Autodesk Inventor part; units mm, degrees
(part 2 of 2)
  arc A608 (10.5835, 25.1123) -> (10.4066, 24.8539) centre (14.8434, 22.0065) ccw
  arc A609 (10.8252, 25.4234) -> (10.5835, 25.1123) centre (15.7615, 21.3378) ccw
  arc A610 (11.147, 25.7878) -> (10.8252, 25.4234) centre (16.6706, 20.5861) ccw
  arc A611 (9.9958, 26.1618) -> (9.6113, 26.2702) centre (4.2393, 6.4866) ccw
  arc A612 (10.0419, 25.6779) -> (9.9958, 26.1618) centre (2.4697, 25.2002) ccw
  arc A613 (10.0547, 25.2841) -> (10.0419, 25.6779) centre (3.647, 25.2741) ccw
  arc A614 (10.4066, 24.8539) -> (10.0459, 24.9711) centre (4.2393, 6.4866) ccw
  arc A615 (10.0459, 24.9711) -> (10.0547, 25.2841) centre (4.7827, 25.2754) ccw
  arc A616 (9.1026, 25.5526) -> (8.9465, 25.2811) centre (13.5931, 22.7906) ccw
  arc A617 (9.3192, 25.8817) -> (9.1026, 25.5526) centre (14.5608, 22.1961) ccw
  arc A618 (9.6113, 26.2702) -> (9.3192, 25.8817) centre (15.526, 21.5179) ccw
  arc A619 (8.4344, 26.5528) -> (8.0426, 26.6307) centre (4.2393, 6.4866) ccw
  arc A620 (8.5183, 26.074) -> (8.4344, 26.5528) centre (1.0069, 25.0037) ccw
  arc A621 (8.5619, 25.6824) -> (8.5183, 26.074) centre (2.1747, 25.1697) ccw
  arc A622 (8.9465, 25.2811) -> (8.5777, 25.3697) centre (4.2393, 6.4866) ccw
  arc A623 (8.5777, 25.3697) -> (8.5619, 25.6824) centre (3.3069, 25.2601) ccw
  arc A624 (7.5917, 25.8754) -> (7.4574, 25.5925) centre (12.285, 23.4742) ccw
  arc A625 (7.7818, 26.2205) -> (7.5917, 25.8754) centre (13.2964, 22.9575) ccw
  arc A626 (8.0426, 26.6307) -> (7.7818, 26.2205) centre (14.3119, 22.3571) ccw
  arc A627 (6.8471, 26.8201) -> (6.4504, 26.867) centre (4.2393, 6.4866) ccw
  arc A628 (6.9683, 26.3493) -> (6.8471, 26.8201) centre (-0.436, 24.693) ccw
  arc A629 (7.0425, 25.9624) -> (6.9683, 26.3493) centre (0.7152, 24.9501) ccw
  arc A630 (7.4574, 25.5925) -> (7.0828, 25.6518) centre (4.2393, 6.4866) ccw
  arc A631 (7.0828, 25.6518) -> (7.0425, 25.9624) centre (1.8368, 25.1291) ccw
  arc A632 (6.0601, 26.0787) -> (5.9484, 25.7861) centre (10.9274, 24.0531) ccw
  arc A633 (6.2226, 26.4376) -> (6.0601, 26.0787) centre (11.9762, 23.6173) ccw
  arc A634 (6.4504, 26.867) -> (6.2226, 26.4376) centre (13.0356, 23.0985) ccw
  arc A635 (5.2437, 26.962) -> (4.8445, 26.9777) centre (4.2393, 6.4866) ccw
  arc A636 (5.4015, 26.5022) -> (5.2437, 26.962) centre (-1.85, 24.27) ccw
  arc A637 (5.5058, 26.1223) -> (5.4015, 26.5022) centre (-0.7225, 24.6167) ccw
  arc A638 (5.9484, 25.7861) -> (5.5703, 25.8158) centre (4.2393, 6.4866) ccw
  arc A639 (5.5703, 25.8158) -> (5.5058, 26.1223) centre (0.3816, 24.8831) ccw
  circle A640 centre (4.2393, 6.4866) radius 18.25
  circle A641 centre (4.2393, 6.4866) radius 6
  circle A642 centre (4.2393, 6.4866) radius 20.5 construction
  circle A643 centre (4.2393, 6.4866) radius 2
  line L0 (4.2393, 6.4866) -> (-6.2776, -1.9776)
  circle A644 centre (-6.2776, -1.9776) radius 1.5
  circle A645 centre (-6.2776, -1.9776) radius 3.5
  circle A646 centre (4.2393, 6.4866) radius 4
  circle A647 centre (12.7036, -4.0303) radius 1.5
  circle A648 centre (12.7036, -4.0303) radius 3.5
  circle A649 centre (14.7563, 14.9509) radius 1.5
  circle A650 centre (14.7563, 14.9509) radius 3.5
  circle A651 centre (-4.225, 17.0036) radius 1.5
  circle A652 centre (-4.225, 17.0036) radius 3.5
  point P0 (0, 0)
  point P1 (0, 0)
  point P2 (4.2393, 28.9866)
  point P3 (2.474, 28.9173)
  point P4 (0.7195, 28.7096)
  point P5 (-1.0132, 28.3649)
  point P6 (-2.7136, 27.8854)
  point P7 (-4.3711, 27.2739)
  point P8 (-5.9755, 26.5343)
  point P9 (-7.5169, 25.671)
  point P10 (-8.9859, 24.6895)
  point P11 (-10.3733, 23.5958)
  point P12 (-11.6706, 22.3965)
  point P13 (-12.8698, 21.0992)
  point P14 (-13.9636, 19.7118)
  point P15 (-14.9451, 18.2428)
  point P16 (-15.8083, 16.7014)
  point P17 (-16.548, 15.097)
  point P18 (-17.1595, 13.4395)
  point P19 (-17.639, 11.7391)
  point P20 (-17.9837, 10.0064)
  point P21 (-18.1913, 8.252)
  point P22 (-18.2607, 6.4866)
  point P23 (-18.1913, 4.7213)
  point P24 (-17.9837, 2.9668)
  point P25 (-17.639, 1.2341)
  point P26 (-17.1595, -0.4663)
  point P27 (-16.548, -2.1238)
  point P28 (-15.8083, -3.7282)
  point P29 (-14.9451, -5.2696)
  point P30 (-13.9636, -6.7385)
  point P31 (-12.8698, -8.126)
  point P32 (-11.6706, -9.4233)
  point P33 (-10.3733, -10.6225)
  point P34 (-8.9859, -11.7163)
  point P35 (-7.5169, -12.6978)
  point P36 (-5.9755, -13.561)
  point P37 (-4.3711, -14.3007)
  point P38 (-2.7136, -14.9121)
  point P39 (-1.0132, -15.3917)
  point P40 (0.7195, -15.7364)
  point P41 (2.474, -15.944)
  point P42 (4.2393, -16.0134)
  point P43 (6.0046, -15.944)
  point P44 (7.7591, -15.7364)
  point P45 (9.4918, -15.3917)
  point P46 (11.1922, -14.9121)
  point P47 (12.8497, -14.3007)
  point P48 (14.4541, -13.561)
  point P49 (15.9955, -12.6978)
  point P50 (17.4645, -11.7163)
  point P51 (18.8519, -10.6225)
  point P52 (20.1492, -9.4233)
  point P53 (21.3484, -8.126)
  point P54 (22.4422, -6.7385)
  point P55 (23.4237, -5.2696)
  point P56 (24.287, -3.7282)
  point P57 (25.0266, -2.1238)
  point P58 (25.6381, -0.4663)
  point P59 (26.1176, 1.2341)
  point P60 (26.4623, 2.9668)
  point P61 (26.6699, 4.7213)
  point P62 (26.7393, 6.4866)
  point P63 (26.6699, 8.252)
  point P64 (26.4623, 10.0064)
  point P65 (26.1176, 11.7391)
  point P66 (25.6381, 13.4395)
  point P67 (25.0266, 15.097)
  point P68 (24.287, 16.7014)
  point P69 (23.4237, 18.2428)
  point P70 (22.4422, 19.7118)
  point P71 (21.3484, 21.0992)
  point P72 (20.1492, 22.3965)
  point P73 (18.8519, 23.5958)
  point P74 (17.4645, 24.6895)
  point P75 (15.9955, 25.671)
  point P76 (14.4541, 26.5343)
  point P77 (12.8497, 27.2739)
  point P78 (11.1922, 27.8854)
  point P79 (9.4918, 28.3649)
  point P80 (7.7591, 28.7096)
  point P81 (6.0046, 28.9173)
  point P82 (6.9688, 26.347)
  point P83 (6.8471, 26.8201)
  point P84 (6.4504, 26.867)
  point P85 (6.2215, 26.4355)
  point P86 (6.059, 26.0761)
  point P87 (5.9484, 25.7861)
  point P88 (5.5703, 25.8158)
  point P89 (5.5065, 26.1196)
  point P90 (5.4022, 26.5)
  point P91 (5.2437, 26.962)
  point P92 (4.8445, 26.9777)
  point P93 (4.6502, 26.5295)
  point P94 (4.5165, 26.1585)
  point P95 (4.4289, 25.8607)
  point P96 (4.0497, 25.8607)
  point P97 (3.9622, 26.1585)
  point P98 (3.8284, 26.5295)
  point P99 (3.6341, 26.9777)
  point P100 (3.2349, 26.962)
  point P101 (3.0764, 26.5)
  point P102 (2.9722, 26.1196)
  point P103 (2.9083, 25.8158)
  point P104 (2.5302, 25.7861)
  point P105 (2.4196, 26.0761)
  point P106 (2.2571, 26.4355)
  point P107 (2.0283, 26.867)
  point P108 (1.6316, 26.8201)
  point P109 (1.5098, 26.347)
  point P110 (1.4357, 25.9597)
  point P111 (1.3958, 25.6518)
  point P112 (1.0212, 25.5925)
  point P113 (0.8882, 25.8729)
  point P114 (0.698, 26.2185)
  point P115 (0.436, 26.6307)
  point P116 (0.0443, 26.5528)
  point P117 (-0.04, 26.0716)
  point P118 (-0.0835, 25.6797)
  point P119 (-0.0991, 25.3697)
  point P120 (-0.4679, 25.2811)
  point P121 (-0.6225, 25.5503)
  point P122 (-0.8392, 25.8798)
  point P123 (-1.1327, 26.2702)
  point P124 (-1.5172, 26.1618)
  point P125 (-1.5635, 25.6755)
  point P126 (-1.5761, 25.2813)
  point P127 (-1.5673, 24.9711)
  point P128 (-1.928, 24.8539)
  point P129 (-2.1032, 25.11)
  point P130 (-2.3451, 25.4216)
  point P131 (-2.6684, 25.7878)
  point P132 (-3.0431, 25.6495)
  point P133 (-3.0511, 25.1611)
  point P134 (-3.0327, 24.7671)
  point P135 (-2.9996, 24.4585)
  point P136 (-3.35, 24.3134)
  point P137 (-3.5448, 24.555)
  point P138 (-3.8104, 24.8466)
  point P139 (-4.1614, 25.1863)
  point P140 (-4.5242, 25.0191)
  point P141 (-4.4938, 24.5315)
  point P142 (-4.4446, 24.1402)
  point P143 (-4.3874, 23.8351)
  point P144 (-4.7253, 23.663)
  point P145 (-4.9385, 23.8886)
  point P146 (-5.2261, 24.1584)
  point P147 (-5.6027, 24.4695)
  point P148 (-5.9512, 24.2743)
  point P149 (-5.8827, 23.7907)
  point P150 (-5.8029, 23.4045)
  point P151 (-5.7219, 23.1048)
  point P152 (-6.0453, 22.9067)
  point P153 (-6.2755, 23.1148)
  point P154 (-6.5834, 23.3613)
  point P155 (-6.9833, 23.6419)
  point P156 (-7.3154, 23.42)
  point P157 (-7.2092, 22.9432)
  point P158 (-7.0993, 22.5644)
  point P159 (-6.9951, 22.272)
  point P160 (-7.3019, 22.0491)
  point P161 (-7.5477, 22.2386)
  point P162 (-7.874, 22.4601)
  point P163 (-8.2947, 22.7085)
  point P164 (-8.6084, 22.4612)
  point P165 (-8.465, 21.9942)
  point P166 (-8.3258, 21.6252)
  point P167 (-8.199, 21.3419)
  point P168 (-8.4873, 21.0956)
  point P169 (-8.7473, 21.2652)
  point P170 (-9.09, 21.4605)
  point P171 (-9.5288, 21.6751)
  point P172 (-9.8221, 21.4039)
  point P173 (-9.6426, 20.9496)
  point P174 (-9.4748, 20.5927)
  point P175 (-9.3261, 20.3202)
  point P176 (-9.5943, 20.0521)
  point P177 (-9.8668, 20.2008)
  point P178 (-10.2237, 20.3685)
  point P179 (-10.678, 20.548)
  point P180 (-10.9492, 20.2547)
  point P181 (-10.7345, 19.8159)
  point P182 (-10.5393, 19.4732)
  point P183 (-10.3697, 19.2133)
  point P184 (-10.616, 18.9249)
  point P185 (-10.8993, 19.0517)
  point P186 (-11.2683, 19.191)
  point P187 (-11.7353, 19.3343)
  point P188 (-11.9826, 19.0206)
  point P189 (-11.7342, 18.6)
  point P190 (-11.5127, 18.2737)
  point P191 (-11.3232, 18.0278)
  point P192 (-11.5461, 17.721)
  point P193 (-11.8385, 17.8252)
  point P194 (-12.2173, 17.9351)
  point P195 (-12.694, 18.0413)
  point P196 (-12.916, 17.7092)
  point P197 (-12.6353, 17.3094)
  point P198 (-12.3889, 17.0015)
  point P199 (-12.1807, 16.7712)
  dimension "d4" = 360
  dimension "d23" = 12
  dimension "d25" = 4
  dimension "d28" = 13.5
  dimension "d29" = 3
  dimension "d30" = 7
  dimension "d31" = 8
  dimension "d34" = 360
  constraints: 1280 point on circle, 652 centre point, 10 coincident, 2 end point, 2659 other
  measures "d23" diameter of A641
  measures "d25" diameter of A643
  measures "d28" distance of L0.start L0.end
  measures "d29" diameter of A644
  measures "d30" diameter of A645
  measures "d31" diameter of A646
extrude "押し出し7" add sketch "スケッチ1" along normal blind 3 contours A1 A2 A635 A636 A637 A639 A638 A632 A633 A634 A627 A628 A629 A631 A630 A624 A625 A626 A619 A620 A621 A623 A622 A616 A617 A618 A611 A612 A613 A615 A614 A608 A609 A610 A603 A604 A605 A607 A606 A600 A601 A602 A595 A596 A597 A599 A598 A592 A593 A594 A587 A588 A589 A591 A590 A584 A585 A586 A579 A580 A581 A583 A582 A576 A577 A578 A571 A572 A573 A575 A574 A568 A569 A570 A563 A564 A565 A567 A566 A560 A561 A562 A555 A556 A557 A559 A558 A552 A553 A554 A547 A548 A549 A551 A550 A544 A545 A546 A539 A540 A541 A543 A542 A536 A537 A538 A531 A532 A533 A535 A534 A528 A529 A530 A523 A524 A525 A527 A526 A520 A521 A522 A515 A516 A517 A519 A518 A512 A513 A514 A507 A508 A509 A511 A510 A504 A505 A506 A499 A500 A501 A503 A502 A496 A497 A498 A491 A492 A493 A495 A494 A488 A489 A490 A483 A484 A485 A487 A486 A480 A481 A482 A475 A476 A477 A479 A478 A472 A473 A474 A467 A468 A469 A471 A470 A464 A465 A466 A459 A460 A461 A463 A462 A456 A457 A458 A451 A452 A453 A455 A454 A448 A449 A450 A443 A444 A445 A447 A446 A440 A441 A442 A435 A436 A437 A439 A438 A432 A433 A434 A427 A428 A429 A431 A430 A424 A425 A426 A419 A420 A421 A423 A422 A416 A417 A418 A411 A412 A413 A415 A414 A408 A409 A410 A403 A404 A405 A407 A406 A400 A401 A402 A395 A396 A397 A399 A398 A392 A393 A394 A387 A388 A389 A391 A390 A384 A385 A386 A379 A380 A381 A383 A382 A376 A377 A378 A371 A372 A373 A375 A374 A368 A369 A370 A363 A364 A365 A367 A366 A360 A361 A362 A355 A356 A357 A359 A358 A352 A353 A354 A347 A348 A349 A351 A350 A344 A345 A346 A339 A340 A341 A343 A342 A336 A337 A338 A331 A332 A333 A335 A334 A328 A329 A330 A323 A324 A325 A327 A326 A320 A321 A322 A315 A316 A317 A319 A318 A312 A313 A314 A307 A308 A309 A311 A310 A304 A305 A306 A299 A300 A301 A303 A302 A296 A297 A298 A291 A292 A293 A295 A294 A288 A289 A290 A283 A284 A285 A287 A286 A280 A281 A282 A275 A276 A277 A279 A278 A272 A273 A274 A267 A268 A269 A271 A270 A264 A265 A266 A259 A260 A261 A263 A262 A256 A257 A258 A251 A252 A253 A255 A254 A248 A249 A250 A243 A244 A245 A247 A246 A240 A241 A242 A235 A236 A237 A239 A238 A232 A233 A234 A227 A228 A229 A231 A230 A224 A225 A226 A219 A220 A221 A223 A222 A216 A217 A218 A211 A212 A213 A215 A214 A208 A209 A210 A203 A204 A205 A207 A206 A200 A201 A202 A195 A196 A197 A199 A198 A192 A193 A194 A187 A188 A189 A191 A190 A184 A185 A186 A179 A180 A181 A183 A182 A176 A177 A178 A171 A172 A173 A175 A174 A168 A169 A170 A163 A164 A165 A167 A166 A160 A161 A162 A155 A156 A157 A159 A158 A152 A153 A154 A147 A148 A149 A151 A150 A144 A145 A146 A139 A140 A141 A143 A142 A136 A137 A138 A131 A132 A133 A135 A134 A128 A129 A130 A123 A124 A125 A127 A126 A120 A121 A122 A115 A116 A117 A119 A118 A112 A113 A114 A107 A108 A109 A111 A110 A104 A105 A106 A99 A100 A101 A103 A102 A96 A97 A98 A91 A92 A93 A95 A94 A88 A89 A90 A83 A84 A85 A87 A86 A80 A81 A82 A75 A76 A77 A79 A78 A72 A73 A74 A67 A68 A69 A71 A70 A64 A65 A66 A59 A60 A61 A63 A62 A56 A57 A58 A51 A52 A53 A55 A54 A48 A49 A50 A43 A44 A45 A47 A46 A40 A41 A42 A35 A36 A37 A39 A38 A32 A33 A34 A27 A28 A29 A31 A30 A24 A25 A26 A19 A20 A21 A23 A22 A16 A17 A18 A11 A12 A13 A15 A14 A8 A9 A10 A7 A5 A4 A3 A6 A0 | A640
extrude "押し出し8" add sketch "スケッチ1" along normal blind 2.2 contours A645 | A648 | A650 | A652
sketch "スケッチ2" plane through (0, 0, 3) normal (0, 0, 1) x (1, 0, 0)
  circle A0 centre (4.2393, 6.4866) radius 6 projected
  circle A1 centre (4.2393, 6.4866) radius 18.25
  point P0 (0, 0)
  dimension "d38" = 36.5
  constraints: 1 centre point, 1 coincident
  measures "d38" diameter of A1
extrude "押し出し9" cut sketch "スケッチ2" against normal blind 0.6 contours A0 | A1
sketch "スケッチ3" plane through (0, 0, 0) normal (0, 0, -1) x (-1, 0, 0)
  circle A0 centre (-4.2393, 6.4866) radius 6 projected
  circle A1 centre (-4.2393, 6.4866) radius 18.25
  point P0 (0, 0)
  dimension "d41" = 36.5
  constraints: 1 centre point, 1 coincident
  measures "d41" diameter of A1
extrude "押し出し10" cut sketch "スケッチ3" against normal blind 0.6
